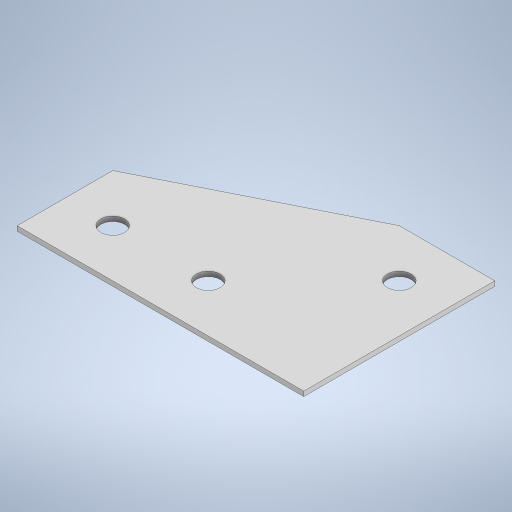
# Autodesk Inventor part: Угол 80х40
Saved by Autodesk Inventor 2023 (Build 270158000, 158)
## iProperties
Created: 2022-05-05
Part Number: Угол 80х40
Material: Типовые
Document SubType Name: Modeling
Designer: avkap
Density: 1 g/cm^3
Appearance: По умолчанию
Author: avkap
Autodesk Inventor part; units mm, degrees
ref_plane "YZ Plane" through (0, 0, 0) normal (1, 0, 0) x (0, 1, 0)
ref_plane "XZ Plane" through (0, 0, 0) normal (0, 1, 0) x (-1, 0, 0)
ref_plane "XY Plane" through (0, 0, 0) normal (0, 0, 1) x (1, 0, 0)
sketch "Эскиз1" plane through (0, 0, 0) normal (0, 1, 0) x (-1, 0, 0)
  line L0 (0, 0) -> (80, 0)
  line L1 (80, 0) -> (80, -80)
  line L2 (80, -80) -> (0, -80)
  line L3 (0, -80) -> (0, 0)
  line L4 (80, 0) -> (80, -40)
  line L5 (80, -20) -> (60, -20)
  line L6 (40, -80) -> (0, -80)
  line L7 (20, -80) -> (20, -60)
  circle A0 centre (60, -20) radius 5
  circle A1 centre (20, -60) radius 5
  line L8 (80, 0) -> (120, 0)
  line L9 (120, 0) -> (120, -40)
  line L10 (120, -40) -> (80, -40)
  line L11 (80, -40) -> (80, 0)
  line L12 (0, -80) -> (40, -80)
  line L13 (40, -80) -> (120, -40)
  line L14 (80, -20) -> (100, -20)
  circle A2 centre (100, -20) radius 5
  dimension "d0" = 80
  dimension "d1" = 80
  dimension "d2" = 40
  dimension "d3" = 20
  dimension "d4" = 20
  dimension "d5" = 10
  dimension "d6" = 10
  dimension "d7" = 40
  dimension "d8" = 40
  dimension "d9" = 40
  dimension "d10" = 10
  constraints: 30 end point, 4 horizontal, 4 midpoint, 4 parallel, 3 centre point, 2 coincident, 2 collinear, 2 perpendicular, 1 vertical
  measures "d0" distance of L1.end L2.end
  measures "d1" distance of L0.end L1.end
  measures "d2" distance of L0.end L4.end
  measures "d3" distance of L5.start L5.end
  measures "d4" distance of L7.start L7.end
  measures "d5" diameter of A0
  measures "d6" diameter of A1
  measures "d7" distance of L9.end L10.end
  measures "d8" distance of L8.end L9.end
  measures "d9" distance of L2.end L6.start
  measures "d10" diameter of A2
extrude "Выдавливание1" add sketch "Эскиз1" along normal blind 2 contours L0 L1 L13 L2 L3 | L8 L9 L10 L1 | L10 L13 L1
